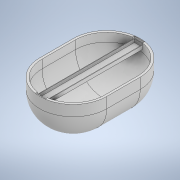
# Autodesk Inventor part: lid
Saved by Autodesk Inventor 2021 (Build 250183000, 183)
## iProperties
Created: 2021-01-26
Part Number: lid
Material: Generic
Document SubType Name: Modeling
Designer: Kayla
Density: 1 g/cm^3
Appearance: Default
Author: Kayla
Autodesk Inventor part; units mm, degrees
ref_plane "YZ Plane" through (0, 0, 0) normal (1, 0, 0) x (0, 1, 0)
ref_plane "XZ Plane" through (0, 0, 0) normal (0, 1, 0) x (-1, 0, 0)
ref_plane "XY Plane" through (0, 0, 0) normal (0, 0, 1) x (1, 0, 0)
sketch "Sketch1" plane through (0, 0, 0) normal (0, 1, 0) x (-1, 0, 0)
  line L0 (0, 0) -> (0, -60) construction
  line L1 (-60, 0) -> (-60, -60)
  line L2 (60, -60) -> (60, 0)
  arc A0 (60, 0) -> (-60, 0) centre (0, 0) ccw
  arc A1 (-60, -60) -> (60, -60) centre (0, -60) ccw
  line L3 (56, 0) -> (56, -60)
  arc A2 (-56, -60) -> (56, -60) centre (0, -60) ccw
  line L4 (-56, -60) -> (-56, 0)
  arc A3 (56, 0) -> (-56, 0) centre (0, 0) ccw
  point P0 (0, -30)
  dimension "d0" = 60
  dimension "d1" = 60
  dimension "d4" = 4
  constraints: 12 end point, 8 point on circle, 4 centre point, 4 tangent, 2 parallel, 1 midpoint, 1 vertical, 3 other
  measures "d0" distance of L2.start L2.end
  measures "d1" radius of A0
  measures "d4" radial gap between concentric circles of A1 A2
extrude "Extrusion2" add sketch "Sketch1" along normal blind 70
extrude "Extrusion3" add sketch "Sketch1" along normal blind 4 contours L3 A2 L4 A3
fillet "Fillet1" radius 50.8 8 edges at (0, 4, 56) (-56, 4, -30) (0, 4, -116) (56, 4, -30) (0, 0, 60) (60, 0, -30) (0, 0, -120) (-60, 0, -30)
sketch "Sketch5" plane through (0, 70, 0) normal (0, 1, 0) x (1, 0, 0)
  line L0 (-9, 118.645) -> (9, 118.645)
  line L1 (9, 118.645) -> (9, -58.355)
  line L2 (9, -58.355) -> (-9, -58.355)
  line L3 (-9, -58.355) -> (-9, 118.645)
  point P0 (0, 0)
  dimension "d11" = 177
  dimension "d12" = 18
  dimension "d13" = 9
  constraints: 8 end point, 2 parallel, 1 horizontal, 1 perpendicular
  measures "d11" distance of L0.end L1.end
  measures "d12" distance of L1.end L2.end
  measures "d13" distance from line of L3 point (0, 0)
extrude "Extrusion4" add sketch "Sketch5" against normal blind 10
extrude "Extrusion5" cut sketch "Sketch5" against normal blind 9
sketch "Sketch6" plane through (0, 61, 0) normal (0, 1, 0) x (1, 0, 0)
  line L0 (-9, 118.6362) -> (9, 118.6362)
  line L1 (9, 118.6362) -> (9, -58.3638)
  line L2 (9, -58.3638) -> (-9, -58.3638)
  line L3 (-9, -58.3638) -> (-9, 118.6362)
  line L4 (-8, 117.6362) -> (8, 117.6362)
  line L5 (8, 117.6362) -> (8, -57.3638)
  line L6 (8, -57.3638) -> (-8, -57.3638)
  line L7 (-8, -57.3638) -> (-8, 117.6362)
  point P0 (0, 0)
  dimension "d19" = 177
  dimension "d20" = 18
  dimension "d21" = 9
  dimension "d22" = 1
  constraints: 16 end point, 4 parallel, 2 perpendicular, 1 horizontal, 3 other
  measures "d19" distance of L2.end L0.start
  measures "d20" distance of L0.start L0.end
  measures "d21" distance from line of L3 point (0, 0)
  measures "d22" distance between parallel lines of L3 L7
extrude "Extrusion6" add sketch "Sketch6" along normal blind 5.5
body "Solid2"
